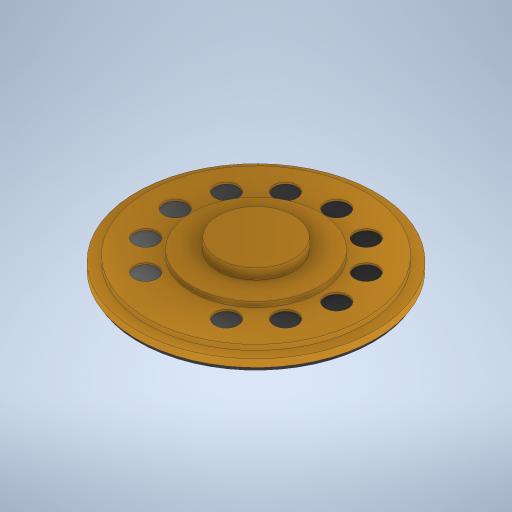
# Autodesk Inventor part: speaker
Saved by Autodesk Inventor 2023 (Build 270158000, 158)
## iProperties
Created: 2022-06-06
Part Number: speaker
Material: 일반
Document SubType Name: Modeling
Designer: fly01
Density: 1 g/cm^3
Appearance: 기본값
Author: fly01
Autodesk Inventor part; units mm, degrees
ref_plane "YZ Plane" through (0, 0, 0) normal (1, 0, 0) x (0, 1, 0)
ref_plane "XZ Plane" through (0, 0, 0) normal (0, 1, 0) x (-1, 0, 0)
ref_plane "XY Plane" through (0, 0, 0) normal (0, 0, 1) x (1, 0, 0)
sketch "스케치1" plane through (0, 0, 0) normal (0, 0, 1) x (1, 0, 0)
  line L0 (0, 0) -> (0, 32.9047)
  line L1 (0, 0) -> (28.5, 0)
  line L2 (28.5, 0) -> (28.5, 2.8)
  line L3 (28.5, 2.8) -> (26.075, 2.8)
  line L4 (26.075, 2.8) -> (26.075, 4.05)
  line L5 (26.075, 4.05) -> (0, 4.05)
  line L6 (28.5, 2.8) -> (28.5, 1)
  line L7 (28.5, 1) -> (27.9, 1)
  line L8 (27.9, 1) -> (27.9, 0)
  line L9 (27.9, 0) -> (26.3, 0)
  line L10 (26.3, 0) -> (26.3, 1.75)
  line L11 (-6.25, 2) -> (6.25, 2)
  arc A0 (-6.25, 2) -> (6.25, 2) centre (0, 21.0312) ccw
  line L12 (0, 1) -> (0, 2)
  arc A1 (6.25, 2) -> (26.3, 1.75) centre (18.9509, 216.4804) ccw
  line L13 (26.3, 1.75) -> (26.3, 1.95)
  line L14 (26.3, 1.95) -> (0, 2.4617)
  line L15 (26.3, 1.95) -> (26.3, 2.4617)
  line L16 (26.3, 2.4617) -> (25.7694, 2.4617)
  line L17 (25.7694, 2.4617) -> (25.7694, 3.656)
  line L18 (25.7694, 3.656) -> (0, 3.656)
  point P0 (0, 1)
  dimension "d1" = 28.5
  dimension "d2" = 2.8
  dimension "d3" = 26.075
  dimension "d4" = 1.25
  dimension "d5" = 1.8
  dimension "d6" = 0.6
  dimension "d7" = 1.6
  dimension "d8" = 1.75
  dimension "d9" = 12.5
  dimension "d10" = 0.8
  dimension "d11" = 1
  dimension "d19" = 0.2
  constraints: 38 end point, 11 perpendicular, 7 point on line, 5 point on circle, 2 centre point, 2 horizontal, 2 vertical, 1 midpoint, 1 vertical alignment
  measures "d1" distance of L0.start L1.end
  measures "d2" distance of L1.end L2.end
  measures "d3" distance of L4.end L5.end
  measures "d4" distance of L3.end L4.end
  measures "d5" distance of L2.end L6.end
  measures "d6" distance of L6.end L7.end
  measures "d7" distance of L8.end L9.end
  measures "d8" distance of L9.end L10.end
  measures "d9" distance of L11.start L11.end
  measures "d10" distance between parallel lines of L3 L11
  measures "d11" distance of L12.start L12.end
  measures "d19" distance of L10.end L13.end
revolve "회전1" add sketch "스케치1" angle 360 about axis through (0, 0, 0) along (0, 1, 0) picked at (3.4853, 1.8155) contours L0 L11 A0 | L10 L13 L15 L16 L17 L18 L0 L5 L4 L3 L2 L7 L8 L1 | L0 L14 L13 A1 L11
sketch "스케치2" plane through (0, 4.05, 0) normal (0, 1, 0) x (1, 0, 0)
  circle A0 centre (0, 0) radius 15.275
  dimension "d13" = 30.55
  constraints: 1 centre point, 1 coincident
  measures "d13" diameter of A0
extrude "돌출1" add sketch "스케치2" along normal blind 1.2
sketch "스케치3" plane through (0, 5.25, 0) normal (0, 1, 0) x (1, 0, 0)
  circle A0 centre (0, 0) radius 9
  dimension "d16" = 18
  constraints: 1 centre point, 1 coincident
  measures "d16" diameter of A0
extrude "돌출2" add sketch "스케치3" along normal blind 2.5
sketch "스케치4" plane through (0, 4.05, 0) normal (0, 1, 0) x (1, 0, 0)
  point P0 (0, 0)
sketch "스케치5" plane through (0, 4.05, 0) normal (0, 1, 0) x (1, 0, 0)
  circle A0 centre (0, 19.25) radius 2.75
  line L0 (0, 19.25) -> (0, 0)
  dimension "d20" = 5.5
  dimension "d21" = 19.25
  constraints: 2 end point, 1 centre point, 1 vertical
  measures "d20" diameter of A0
  measures "d21" distance of L0.start L0.end
extrude "돌출3" cut sketch "스케치5" against normal blind 0.5
pattern_circular "원형 패턴1" count 12 over 360 about axis through (0, 4.05, 0) along (0, 1, 0) of "돌출3"
sketch "스케치6" plane through (0, 4.05, 0) normal (0, 1, 0) x (1, 0, 0)
  circle A0 centre (0, -19.25) radius 2.75 projected
  point P0 (0, 0)
extrude "돌출4" add sketch "스케치6" against normal blind 0.5
